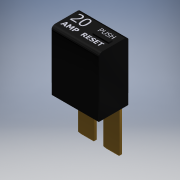
# Autodesk Inventor part: VB3-A30-F57
Saved by Autodesk Inventor 2017.1 (Build 211199000, 199)
## iProperties
Category: Bag #3
Company: Autodesk Inc.
Created: 2016-12-24
Part Number: VB3-A30-F57
Document SubType Name: Modeling
Designer: Autodesk Inc.
Density: 1 g/cm^3
Material: Generic
Catalog Web Link: www.snapaction.net
Vendor: Snap Action Inc.
Appearance: Glossy - Black
Author: Autodesk Inc.
Keywords: Gray Tote
Autodesk Inventor part; units mm, degrees
note: some values were not read from the file. Chosen so that the rebuilt part matches the saved one: direction of "Emboss1"; direction of "Emboss2".
sketch "Sketch1" plane through (0, 0, 0) normal (0, 0, 1) x (1, 0, 0)
  line L0 (0, 0) -> (15.748, 0)
  line L1 (15.748, 0) -> (15.748, 9.906)
  line L2 (15.748, 9.906) -> (0, 9.906)
  line L3 (0, 9.906) -> (0, 0)
  dimension "d0" = 15.748
  dimension "d1" = 9.906
  constraints: 8 end point, 2 parallel, 1 horizontal, 1 perpendicular
  measures "d0" distance of L1.end L2.end
  measures "d1" distance of L0.end L1.end
extrude "Extrusion1" add sketch "Sketch1" against normal blind 19.812
fillet "Fillet1" radius 0.254 8 edges at (0, 0, -9.906) (15.748, 0, -9.906) (15.748, 9.906, -9.906) (0, 9.906, -9.906) (7.874, 0, -19.812) (7.874, 9.906, -19.812) (15.748, 4.953, -19.812) (0, 4.953, -19.812)
fillet "Fillet1" radius 1.27 2 edges at (7.874, 0, 0) (7.874, 9.906, 0)
sketch "Sketch2" plane through (0, 0, -19.812) normal (0, 0, -1) x (-1, 0, 0)
  line L0 (-1.0033, 8.6678) -> (-6.3881, 8.6677)
  line L1 (-6.3881, 8.6677) -> (-6.3881, 7.8803)
  line L2 (-6.3881, 7.8803) -> (-1.0033, 7.8803)
  line L3 (-1.0033, 7.8803) -> (-1.0033, 8.6678)
  line L4 (-0.254, 9.906) -> (-15.494, 9.906) projected
  line L5 (-0.254, 0.254) -> (-15.494, 0.254) projected
  line L6 (-15.494, 9.652) -> (-0.254, 9.652) projected
  line L7 (-7.874, 0.254) -> (-7.874, 9.652) construction
  point P0 (0, 0)
  dimension "d6" = 5.3848
  dimension "d8" = 0.7874
  dimension "d13" = 1.4859
  constraints: 10 end point, 2 midpoint, 2 parallel, 1 horizontal, 1 perpendicular
  measures "d6" distance of L1.end L2.end
  measures "d8" distance of L2.end L0.start
  measures "d13" distance between parallel lines of L7 L1
extrude "Extrusion3" add sketch "Sketch2" along normal blind 14.478
sketch "Sketch3" plane through (6.3881, 7.8803, -19.812) normal (1, 0, 0) x (0, 0, -1)
  line L0 (14.478, 0) -> (14.478, 0.7874) projected
  line L1 (0, 0.7874) -> (14.478, 0.7874) projected
  line L2 (0, 0) -> (14.478, 0) projected
  line L3 (13.8941, 0) -> (14.478, 0.3937)
  line L4 (13.8941, 0.7874) -> (14.478, 0.3937)
  point P0 (-19.812, -7.8803)
  constraints: 4 end point, 2 point on line, 1 midpoint
extrude "Extrusion4" cut sketch "Sketch3" against normal up to next
sketch "Sketch4" plane through (1.0033, 7.8803, -19.812) normal (0, -1, 0) x (1, 0, 0)
  line L0 (5.3848, -14.478) -> (0, -14.478) projected
  line L1 (0, -13.8941) -> (0.5839, -14.478)
  line L2 (5.3848, -13.8941) -> (4.8009, -14.478)
  line L3 (0, -13.8941) -> (0, -14.478)
  line L4 (4.8009, -14.478) -> (5.3848, -14.478)
  line L5 (5.3848, -13.8941) -> (5.3848, -14.478)
  point P0 (-1.0033, 19.812)
  dimension "d18" = 0.5839
  dimension "d19" = 0.5839
  dimension "d20" = 0.5839
  constraints: 10 end point, 3 perpendicular, 2 point on line, 1 collinear
  measures "d18" distance of L0.end L1.start
  measures "d19" distance of L1.end L0.end
  measures "d20" distance of L0.start L2.end
extrude "Extrusion5" cut sketch "Sketch4" against normal through all
ref_plane "Work Plane1" through (7.874, 1.27, 0) normal (1, 0, 0) x (0, 0, -1)
mirror "Mirror1" about plane through (7.874, 1.27, 0) normal (1, 0, 0) of "Extrusion3", "Extrusion4", "Extrusion5"
sketch "Sketch5" plane through (0, 0, 0) normal (0, 0, 1) x (1, 0, 0)
  line L0 (15.748, 1.27) -> (15.748, 8.636) projected
  line L1 (9.3525, 4.3197) -> (14.6865, 4.3197)
  line L2 (14.6865, 4.3197) -> (14.6865, 5.5863)
  line L3 (14.6865, 5.5863) -> (9.3525, 5.5863)
  line L4 (9.3525, 5.5863) -> (9.3525, 4.3197)
  point P0 (0, 0)
  point P1 (14.6865, 4.953)
  point P2 (15.748, 4.953)
  dimension "d23" = 5.334
  constraints: 8 end point, 2 midpoint, 2 parallel, 1 horizontal, 1 horizontal alignment, 1 perpendicular
  measures "d23" distance of L2.end L3.end
extrude "Extrusion6" add sketch "Sketch5" along normal blind 0.508
ref_plane "Work Plane2" through (0, 0, 4.7625) normal (0, 0, 1) x (1, 0, 0)
sketch "Sketch6" plane through (0, 0, 4.7625) normal (0, 0, 1) x (1, 0, 0)
  line L0 (0.8788, 8.3471) -> (9.0578, 8.3471) construction
  line L1 (9.0578, 8.3471) -> (9.0578, -5.6048) construction
  line L2 (9.0578, -5.6048) -> (0.8788, -5.6048) construction
  line L3 (0.8788, -5.6048) -> (0.8788, 8.3471) construction
  line L4 (3.156, 4.9755) -> (1.1197, 4.9755)
  line L5 (1.1197, 4.9755) -> (1.1197, 5.4438)
  spline S0 degree 2 poles (1.1197, 5.4438) (1.3391, 5.6498) (1.7298, 6.0325) (1.9171, 6.2385) knots 0 0 0 1 2 2 2
  spline S1 degree 2 poles (1.9171, 6.2385) (2.2944, 6.6533) (2.57, 7.151) (2.57, 7.4159) knots 0 0 0 1 2 2 2
  spline S2 degree 2 poles (2.57, 7.4159) (2.57, 7.555) (2.4843, 7.7638) (2.4067, 7.8307) knots 0 0 0 1 2 2 2
  spline S3 degree 2 poles (2.4067, 7.8307) (2.3291, 7.8976) (2.1258, 7.9644) (2.0027, 7.9644) knots 0 0 0 1 2 2 2
  spline S4 degree 2 poles (2.0027, 7.9644) (1.885, 7.9644) (1.6441, 7.9056) (1.5344, 7.8601) knots 0 0 0 1 2 2 2
  spline S5 degree 2 poles (1.5344, 7.8601) (1.4408, 7.8226) (1.2668, 7.7156) (1.2133, 7.6781) knots 0 0 0 1 2 2 2
  line L6 (1.2133, 7.6781) -> (1.1892, 7.6781)
  line L7 (1.1892, 7.6781) -> (1.1892, 8.1491)
  spline S6 degree 2 poles (1.1892, 8.1491) (1.3257, 8.216) (1.8154, 8.3471) (2.0348, 8.3471) knots 0 0 0 1 2 2 2
  spline S7 degree 2 poles (2.0348, 8.3471) (2.4977, 8.3471) (3.0195, 7.8574) (3.0195, 7.44) knots 0 0 0 1 2 2 2
  spline S8 degree 2 poles (3.0195, 7.44) (3.0195, 7.2446) (2.9285, 6.9182) (2.8483, 6.779) knots 0 0 0 1 2 2 2
  spline S9 degree 2 poles (2.8483, 6.779) (2.768, 6.6345) (2.5352, 6.3509) (2.4067, 6.2144) knots 0 0 0 1 2 2 2
  spline S10 degree 2 poles (2.4067, 6.2144) (2.198, 5.987) (1.6869, 5.5) (1.5344, 5.3582) knots 0 0 0 1 2 2 2
  line L8 (1.5344, 5.3582) -> (3.156, 5.3582)
  line L9 (3.156, 5.3582) -> (3.156, 4.9755)
  spline S11 degree 2 poles (5.6526, 6.6265) (5.6526, 5.7381) (5.1361, 4.9059) (4.5983, 4.9059) knots 0 0 0 1 2 2 2
  spline S12 degree 2 poles (4.5983, 4.9059) (4.0524, 4.9059) (3.5413, 5.7542) (3.5413, 6.6238) knots 0 0 0 1 2 2 2
  spline S13 degree 2 poles (3.5413, 6.6238) (3.5413, 7.5176) (4.0577, 8.3444) (4.5983, 8.3444) knots 0 0 0 1 2 2 2
  spline S14 degree 2 poles (4.5983, 8.3444) (5.1415, 8.3444) (5.6526, 7.4881) (5.6526, 6.6265) knots 0 0 0 1 2 2 2
  spline S15 degree 2 poles (5.0853, 5.6204) (5.1495, 5.7836) (5.203, 6.2867) (5.203, 6.6265) knots 0 0 0 1 2 2 2
  spline S16 degree 2 poles (5.203, 6.6265) (5.203, 6.9664) (5.1495, 7.4667) (5.0826, 7.6353) knots 0 0 0 1 2 2 2
  spline S17 degree 2 poles (5.0826, 7.6353) (5.0157, 7.8039) (4.7829, 7.9778) (4.5983, 7.9778) knots 0 0 0 1 2 2 2
  spline S18 degree 2 poles (4.5983, 7.9778) (4.4136, 7.9778) (4.1755, 7.8039) (4.1059, 7.63) knots 0 0 0 1 2 2 2
  spline S19 degree 2 poles (4.1059, 7.63) (4.039, 7.4614) (3.9909, 6.9476) (3.9909, 6.6238) knots 0 0 0 1 2 2 2
  spline S20 degree 2 poles (3.9909, 6.6238) (3.9909, 6.276) (4.0337, 5.8104) (4.1032, 5.6284) knots 0 0 0 1 2 2 2
  spline S21 degree 2 poles (4.1032, 5.6284) (4.1675, 5.4572) (4.4056, 5.2725) (4.5983, 5.2725) knots 0 0 0 1 2 2 2
  spline S22 degree 2 poles (4.5983, 5.2725) (4.7802, 5.2725) (5.0184, 5.4465) (5.0853, 5.6204) knots 0 0 0 1 2 2 2
  line L10 (0.8721, 2.0545) -> (1.4301, 3.7055)
  line L11 (1.4301, 3.7055) -> (1.8823, 3.7055)
  line L12 (1.8823, 3.7055) -> (2.4402, 2.0545)
  line L13 (2.4402, 2.0545) -> (2.0134, 2.0545)
  line L14 (2.0134, 2.0545) -> (1.9104, 2.3917)
  line L15 (1.9104, 2.3917) -> (1.3913, 2.3917)
  line L16 (1.3913, 2.3917) -> (1.2869, 2.0545)
  line L17 (1.2869, 2.0545) -> (0.8721, 2.0545)
  line L18 (1.8194, 2.6914) -> (1.6508, 3.2372)
  line L19 (1.6508, 3.2372) -> (1.4809, 2.6914)
  line L20 (1.4809, 2.6914) -> (1.8194, 2.6914)
  line L21 (4.2905, 2.0545) -> (3.8785, 2.0545)
  line L22 (3.8785, 2.0545) -> (3.8785, 3.1489)
  line L23 (3.8785, 3.1489) -> (3.5788, 2.4425)
  line L24 (3.5788, 2.4425) -> (3.2951, 2.4425)
  line L25 (3.2951, 2.4425) -> (2.9954, 3.1489)
  line L26 (2.9954, 3.1489) -> (2.9954, 2.0545)
  line L27 (2.9954, 2.0545) -> (2.6048, 2.0545)
  line L28 (2.6048, 2.0545) -> (2.6048, 3.7055)
  line L29 (2.6048, 3.7055) -> (3.0824, 3.7055)
  line L30 (3.0824, 3.7055) -> (3.449, 2.8907)
  line L31 (3.449, 2.8907) -> (3.8129, 3.7055)
  line L32 (3.8129, 3.7055) -> (4.2905, 3.7055)
  line L33 (4.2905, 3.7055) -> (4.2905, 2.0545)
  spline S23 degree 2 poles (5.9027, 3.1851) (5.9027, 3.07) (5.8292, 2.8613) (5.7609, 2.7917) knots 0 0 0 1 2 2 2
  spline S24 degree 2 poles (5.7609, 2.7917) (5.7195, 2.7476) (5.6178, 2.6753) (5.5576, 2.6499) knots 0 0 0 1 2 2 2
  spline S25 degree 2 poles (5.5576, 2.6499) (5.496, 2.6245) (5.3529, 2.595) (5.2646, 2.595) knots 0 0 0 1 2 2 2
  line L34 (5.2646, 2.595) -> (5.0478, 2.595)
  line L35 (5.0478, 2.595) -> (5.0478, 2.0545)
  line L36 (5.0478, 2.0545) -> (4.6331, 2.0545)
  line L37 (4.6331, 2.0545) -> (4.6331, 3.7055)
  line L38 (4.6331, 3.7055) -> (5.2739, 3.7055)
  spline S26 degree 2 poles (5.2739, 3.7055) (5.4157, 3.7055) (5.6231, 3.6533) (5.7074, 3.5971) knots 0 0 0 1 2 2 2
  spline S27 degree 2 poles (5.7074, 3.5971) (5.8011, 3.5343) (5.9027, 3.3282) (5.9027, 3.1851) knots 0 0 0 1 2 2 2
  spline S28 degree 2 poles (5.4773, 3.1744) (5.4773, 3.2453) (5.4104, 3.3456) (5.3649, 3.3643) knots 0 0 0 1 2 2 2
  spline S29 degree 2 poles (5.3649, 3.3643) (5.306, 3.3898) (5.199, 3.3978) (5.1067, 3.3978) knots 0 0 0 1 2 2 2
  line L39 (5.1067, 3.3978) -> (5.0478, 3.3978)
  line L40 (5.0478, 3.3978) -> (5.0478, 2.9028)
  line L41 (5.0478, 2.9028) -> (5.0772, 2.9028)
  spline S30 degree 2 poles (5.0772, 2.9028) (5.1348, 2.9028) (5.2391, 2.9054) (5.2779, 2.9121) knots 0 0 0 1 2 2 2
  spline S31 degree 2 poles (5.2779, 2.9121) (5.3114, 2.9175) (5.385, 2.9496) (5.405, 2.9697) knots 0 0 0 1 2 2 2
  spline S32 degree 2 poles (5.405, 2.9697) (5.4479, 3.0098) (5.4773, 3.0994) (5.4773, 3.1744) knots 0 0 0 1 2 2 2
  point P0 (0, 0)
  constraints: 2 other
emboss "Emboss1" sketch "Sketch6" operation cut depth 0.0025 direction (0, 0, -1)
ref_plane "Work Plane3" through (0, 0, 3.175) normal (0, 0, 1) x (1, 0, 0)
sketch "Sketch7" plane through (0, 0, 3.175) normal (0, 0, 1) x (1, 0, 0)
  line L0 (8.4572, 7.7891) -> (13.9877, 7.7891) construction
  line L1 (13.9877, 7.7891) -> (13.9877, 2.1169) construction
  line L2 (13.9877, 2.1169) -> (8.4572, 2.1169) construction
  line L3 (8.4572, 2.1169) -> (8.4572, 7.7891) construction
  line L4 (15.748, 1.27) -> (15.748, 8.636) projected
  spline S0 degree 2 poles (9.9924, 7.3025) (9.9924, 7.2037) (9.922, 7.0259) (9.8591, 6.9641) knots 0 0 0 1 2 2 2
  spline S1 degree 2 poles (9.8591, 6.9641) (9.78, 6.8863) (9.5664, 6.806) (9.4033, 6.806) knots 0 0 0 1 2 2 2
  line L5 (9.4033, 6.806) -> (9.2317, 6.806)
  line L6 (9.2317, 6.806) -> (9.2317, 6.2379)
  line L7 (9.2317, 6.2379) -> (9.0291, 6.2379)
  line L8 (9.0291, 6.2379) -> (9.0291, 7.7619)
  line L9 (9.0291, 7.7619) -> (9.412, 7.7619)
  spline S2 degree 2 poles (9.412, 7.7619) (9.5478, 7.7619) (9.738, 7.7175) (9.8109, 7.6668) knots 0 0 0 1 2 2 2
  spline S3 degree 2 poles (9.8109, 7.6668) (9.8961, 7.6088) (9.9924, 7.4297) (9.9924, 7.3025) knots 0 0 0 1 2 2 2
  spline S4 degree 2 poles (9.7812, 7.2963) (9.7812, 7.3754) (9.7269, 7.4915) (9.6713, 7.5285) knots 0 0 0 1 2 2 2
  spline S5 degree 2 poles (9.6713, 7.5285) (9.6232, 7.5606) (9.4947, 7.5866) (9.3996, 7.5866) knots 0 0 0 1 2 2 2
  line L10 (9.3996, 7.5866) -> (9.2317, 7.5866)
  line L11 (9.2317, 7.5866) -> (9.2317, 6.9789)
  line L12 (9.2317, 6.9789) -> (9.37, 6.9789)
  spline S6 degree 2 poles (9.37, 6.9789) (9.4935, 6.9789) (9.6454, 7.0185) (9.6948, 7.0703) knots 0 0 0 1 2 2 2
  spline S7 degree 2 poles (9.6948, 7.0703) (9.7405, 7.116) (9.7812, 7.2235) (9.7812, 7.2963) knots 0 0 0 1 2 2 2
  spline S8 degree 2 poles (10.7174, 6.2058) (10.5828, 6.2058) (10.3827, 6.2762) (10.3123, 6.3466) knots 0 0 0 1 2 2 2
  spline S9 degree 2 poles (10.3123, 6.3466) (10.232, 6.4257) (10.1666, 6.648) (10.1666, 6.811) knots 0 0 0 1 2 2 2
  line L13 (10.1666, 6.811) -> (10.1666, 7.7619)
  line L14 (10.1666, 7.7619) -> (10.3691, 7.7619)
  line L15 (10.3691, 7.7619) -> (10.3691, 6.811)
  spline S10 degree 2 poles (10.3691, 6.811) (10.3691, 6.7048) (10.3963, 6.5615) (10.4346, 6.5035) knots 0 0 0 1 2 2 2
  spline S11 degree 2 poles (10.4346, 6.5035) (10.4753, 6.4417) (10.6161, 6.3787) (10.7174, 6.3787) knots 0 0 0 1 2 2 2
  spline S12 degree 2 poles (10.7174, 6.3787) (10.8125, 6.3787) (10.9607, 6.4417) (11.0014, 6.5035) knots 0 0 0 1 2 2 2
  spline S13 degree 2 poles (11.0014, 6.5035) (11.0397, 6.5615) (11.0669, 6.7035) (11.0669, 6.806) knots 0 0 0 1 2 2 2
  line L16 (11.0669, 6.806) -> (11.0669, 7.7619)
  line L17 (11.0669, 7.7619) -> (11.2694, 7.7619)
  line L18 (11.2694, 7.7619) -> (11.2694, 6.811)
  spline S14 degree 2 poles (11.2694, 6.811) (11.2694, 6.6517) (11.2052, 6.4244) (11.1237, 6.3466) knots 0 0 0 1 2 2 2
  spline S15 degree 2 poles (11.1237, 6.3466) (11.0508, 6.275) (10.8582, 6.2058) (10.7174, 6.2058) knots 0 0 0 1 2 2 2
  spline S16 degree 2 poles (11.9845, 6.2108) (11.819, 6.2108) (11.5868, 6.2799) (11.4843, 6.3293) knots 0 0 0 1 2 2 2
  line L19 (11.4843, 6.3293) -> (11.4843, 6.5837)
  line L20 (11.4843, 6.5837) -> (11.4991, 6.5837)
  spline S17 degree 2 poles (11.4991, 6.5837) (11.5992, 6.4899) (11.8524, 6.3861) (11.9697, 6.3861) knots 0 0 0 1 2 2 2
  spline S18 degree 2 poles (11.9697, 6.3861) (12.1376, 6.3861) (12.3093, 6.5257) (12.3093, 6.6405) knots 0 0 0 1 2 2 2
  spline S19 degree 2 poles (12.3093, 6.6405) (12.3093, 6.7319) (12.2192, 6.8456) (12.1216, 6.874) knots 0 0 0 1 2 2 2
  spline S20 degree 2 poles (12.1216, 6.874) (12.0512, 6.8937) (11.9339, 6.9209) (11.8462, 6.9431) knots 0 0 0 1 2 2 2
  spline S21 degree 2 poles (11.8462, 6.9431) (11.7671, 6.9641) (11.6424, 7.0271) (11.5942, 7.0777) knots 0 0 0 1 2 2 2
  spline S22 degree 2 poles (11.5942, 7.0777) (11.5473, 7.1284) (11.4954, 7.2642) (11.4954, 7.3531) knots 0 0 0 1 2 2 2
  spline S23 degree 2 poles (11.4954, 7.3531) (11.4954, 7.5384) (11.7844, 7.7891) (12.008, 7.7891) knots 0 0 0 1 2 2 2
  spline S24 degree 2 poles (12.008, 7.7891) (12.1364, 7.7891) (12.3637, 7.7385) (12.4612, 7.6903) knots 0 0 0 1 2 2 2
  line L21 (12.4612, 7.6903) -> (12.4612, 7.4482)
  line L22 (12.4612, 7.4482) -> (12.4464, 7.4482)
  spline S25 degree 2 poles (12.4464, 7.4482) (12.3735, 7.5149) (12.1463, 7.6137) (12.0216, 7.6137) knots 0 0 0 1 2 2 2
  spline S26 degree 2 poles (12.0216, 7.6137) (11.8808, 7.6137) (11.7066, 7.4816) (11.7066, 7.3741) knots 0 0 0 1 2 2 2
  spline S27 degree 2 poles (11.7066, 7.3741) (11.7066, 7.2778) (11.8091, 7.163) (11.9055, 7.137) knots 0 0 0 1 2 2 2
  spline S28 degree 2 poles (11.9055, 7.137) (11.9697, 7.1197) (12.1562, 7.0753) (12.2179, 7.0567) knots 0 0 0 1 2 2 2
  spline S29 degree 2 poles (12.2179, 7.0567) (12.3748, 7.0086) (12.5205, 6.8147) (12.5205, 6.6727) knots 0 0 0 1 2 2 2
  spline S30 degree 2 poles (12.5205, 6.6727) (12.5205, 6.5825) (12.4476, 6.4096) (12.3822, 6.3491) knots 0 0 0 1 2 2 2
  spline S31 degree 2 poles (12.3822, 6.3491) (12.3093, 6.2824) (12.1241, 6.2108) (11.9845, 6.2108) knots 0 0 0 1 2 2 2
  line L23 (13.8333, 6.2379) -> (13.6308, 6.2379)
  line L24 (13.6308, 6.2379) -> (13.6308, 6.9839)
  line L25 (13.6308, 6.9839) -> (12.9293, 6.9839)
  line L26 (12.9293, 6.9839) -> (12.9293, 6.2379)
  line L27 (12.9293, 6.2379) -> (12.7267, 6.2379)
  line L28 (12.7267, 6.2379) -> (12.7267, 7.7619)
  line L29 (12.7267, 7.7619) -> (12.9293, 7.7619)
  line L30 (12.9293, 7.7619) -> (12.9293, 7.1642)
  line L31 (12.9293, 7.1642) -> (13.6308, 7.1642)
  line L32 (13.6308, 7.1642) -> (13.6308, 7.7619)
  line L33 (13.6308, 7.7619) -> (13.8333, 7.7619)
  line L34 (13.8333, 7.7619) -> (13.8333, 6.2379)
  line L35 (8.8414, 2.1739) -> (8.3758, 2.1739)
  line L36 (8.3758, 2.1739) -> (7.9522, 2.7334)
  line L37 (7.9522, 2.7334) -> (7.8139, 2.7334)
  line L38 (7.8139, 2.7334) -> (7.8139, 2.1739)
  line L39 (7.8139, 2.1739) -> (7.4335, 2.1739)
  line L40 (7.4335, 2.1739) -> (7.4335, 3.6979)
  line L41 (7.4335, 3.6979) -> (8.0461, 3.6979)
  spline S32 degree 2 poles (8.0461, 3.6979) (8.1733, 3.6979) (8.361, 3.6658) (8.4413, 3.6164) knots 0 0 0 1 2 2 2
  spline S33 degree 2 poles (8.4413, 3.6164) (8.5228, 3.5646) (8.6191, 3.4028) (8.6191, 3.2793) knots 0 0 0 1 2 2 2
  spline S34 degree 2 poles (8.6191, 3.2793) (8.6191, 3.1051) (8.461, 2.8865) (8.3289, 2.8223) knots 0 0 0 1 2 2 2
  line L42 (8.3289, 2.8223) -> (8.8414, 2.1739)
  spline S35 degree 2 poles (8.2264, 3.2311) (8.2264, 3.2891) (8.1819, 3.3719) (8.1313, 3.3941) knots 0 0 0 1 2 2 2
  spline S36 degree 2 poles (8.1313, 3.3941) (8.0955, 3.4089) (8.0078, 3.4176) (7.9423, 3.4176) knots 0 0 0 1 2 2 2
  line L43 (7.9423, 3.4176) -> (7.8139, 3.4176)
  line L44 (7.8139, 3.4176) -> (7.8139, 3.0076)
  line L45 (7.8139, 3.0076) -> (7.9238, 3.0076)
  spline S37 degree 2 poles (7.9238, 3.0076) (8.0028, 3.0076) (8.1152, 3.0273) (8.1535, 3.0582) knots 0 0 0 1 2 2 2
  spline S38 degree 2 poles (8.1535, 3.0582) (8.1906, 3.0878) (8.2264, 3.1669) (8.2264, 3.2311) knots 0 0 0 1 2 2 2
  line L46 (8.955, 2.1739) -> (8.955, 3.6979)
  line L47 (8.955, 3.6979) -> (9.985, 3.6979)
  line L48 (9.985, 3.6979) -> (9.985, 3.4077)
  line L49 (9.985, 3.4077) -> (9.3354, 3.4077)
  line L50 (9.3354, 3.4077) -> (9.3354, 3.1397)
  line L51 (9.3354, 3.1397) -> (9.9344, 3.1397)
  line L52 (9.9344, 3.1397) -> (9.9344, 2.8495)
  line L53 (9.9344, 2.8495) -> (9.3354, 2.8495)
  line L54 (9.3354, 2.8495) -> (9.3354, 2.4642)
  line L55 (9.3354, 2.4642) -> (9.985, 2.4642)
  line L56 (9.985, 2.4642) -> (9.985, 2.1739)
  line L57 (9.985, 2.1739) -> (8.955, 2.1739)
  spline S39 degree 2 poles (10.7149, 2.1468) (10.5395, 2.1468) (10.2753, 2.2147) (10.1616, 2.2641) knots 0 0 0 1 2 2 2
  line L58 (10.1616, 2.2641) -> (10.1616, 2.6272)
  line L59 (10.1616, 2.6272) -> (10.1962, 2.6272)
  spline S40 degree 2 poles (10.1962, 2.6272) (10.3111, 2.5296) (10.5865, 2.4246) (10.7161, 2.4246) knots 0 0 0 1 2 2 2
  spline S41 degree 2 poles (10.7161, 2.4246) (10.7495, 2.4246) (10.8569, 2.4395) (10.8891, 2.4543) knots 0 0 0 1 2 2 2
  spline S42 degree 2 poles (10.8891, 2.4543) (10.9286, 2.4716) (10.9841, 2.5346) (10.9841, 2.5852) knots 0 0 0 1 2 2 2
  spline S43 degree 2 poles (10.9841, 2.5852) (10.9841, 2.6432) (10.894, 2.7149) (10.8322, 2.7309) knots 0 0 0 1 2 2 2
  spline S44 degree 2 poles (10.8322, 2.7309) (10.7544, 2.7519) (10.5778, 2.7877) (10.5, 2.8149) knots 0 0 0 1 2 2 2
  spline S45 degree 2 poles (10.5, 2.8149) (10.3234, 2.8767) (10.1703, 3.0878) (10.1703, 3.2459) knots 0 0 0 1 2 2 2
  spline S46 degree 2 poles (10.1703, 3.2459) (10.1703, 3.4596) (10.5321, 3.7251) (10.8038, 3.7251) knots 0 0 0 1 2 2 2
  spline S47 degree 2 poles (10.8038, 3.7251) (10.9397, 3.7251) (11.2089, 3.6695) (11.3151, 3.6226) knots 0 0 0 1 2 2 2
  line L60 (11.3151, 3.6226) -> (11.3151, 3.2743)
  line L61 (11.3151, 3.2743) -> (11.2818, 3.2743)
  spline S48 degree 2 poles (11.2818, 3.2743) (11.1966, 3.3472) (10.952, 3.4472) (10.8236, 3.4472) knots 0 0 0 1 2 2 2
  spline S49 degree 2 poles (10.8236, 3.4472) (10.773, 3.4472) (10.6939, 3.4324) (10.6495, 3.4126) knots 0 0 0 1 2 2 2
  spline S50 degree 2 poles (10.6495, 3.4126) (10.6136, 3.3966) (10.5618, 3.3324) (10.5618, 3.2929) knots 0 0 0 1 2 2 2
  spline S51 degree 2 poles (10.5618, 3.2929) (10.5618, 3.2336) (10.6445, 3.1656) (10.7631, 3.1385) knots 0 0 0 1 2 2 2
  spline S52 degree 2 poles (10.7631, 3.1385) (10.8397, 3.1212) (10.9817, 3.0878) (11.0632, 3.0594) knots 0 0 0 1 2 2 2
  spline S53 degree 2 poles (11.0632, 3.0594) (11.2213, 3.0014) (11.3756, 2.8087) (11.3756, 2.6506) knots 0 0 0 1 2 2 2
  spline S54 degree 2 poles (11.3756, 2.6506) (11.3756, 2.4234) (11.0187, 2.1468) (10.7149, 2.1468) knots 0 0 0 1 2 2 2
  line L62 (11.572, 2.1739) -> (11.572, 3.6979)
  line L63 (11.572, 3.6979) -> (12.602, 3.6979)
  line L64 (12.602, 3.6979) -> (12.602, 3.4077)
  line L65 (12.602, 3.4077) -> (11.9524, 3.4077)
  line L66 (11.9524, 3.4077) -> (11.9524, 3.1397)
  line L67 (11.9524, 3.1397) -> (12.5514, 3.1397)
  line L68 (12.5514, 3.1397) -> (12.5514, 2.8495)
  line L69 (12.5514, 2.8495) -> (11.9524, 2.8495)
  line L70 (11.9524, 2.8495) -> (11.9524, 2.4642)
  line L71 (11.9524, 2.4642) -> (12.602, 2.4642)
  line L72 (12.602, 2.4642) -> (12.602, 2.1739)
  line L73 (12.602, 2.1739) -> (11.572, 2.1739)
  line L74 (13.1541, 2.1739) -> (13.1541, 3.4077)
  line L75 (13.1541, 3.4077) -> (12.7033, 3.4077)
  line L76 (12.7033, 3.4077) -> (12.7033, 3.6979)
  line L77 (12.7033, 3.6979) -> (13.9877, 3.6979)
  line L78 (13.9877, 3.6979) -> (13.9877, 3.4077)
  line L79 (13.9877, 3.4077) -> (13.5369, 3.4077)
  line L80 (13.5369, 3.4077) -> (13.5369, 2.1739)
  line L81 (13.5369, 2.1739) -> (13.1541, 2.1739)
  point P0 (0, 0)
  point P1 (13.9877, 4.953)
  point P2 (15.748, 4.953)
  constraints: 2 midpoint, 1 horizontal alignment, 2 other
emboss "Emboss2" sketch "Sketch7" operation cut depth 0.0025 direction (0, 0, -1)
equation "\"d19\" = d18"
body "Solid1"
